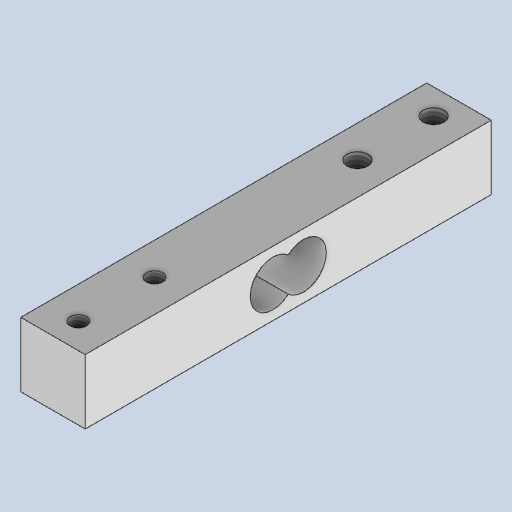
# Autodesk Inventor part: SC133-20kg
Saved by Autodesk Inventor 2022 (Build 260153000, 153)
## iProperties
Part Number: SC133-20kg
Material: 一般
Document SubType Name: Modeling
Designer: Masato Kubotera
Density: 1 g/cm^3
Appearance: 既定
Catalog Web Link: https://akizukidenshi.com/catalog/g/gP-12034/
Description: ReadyMade
Mass: 10.9137 g
Surface Area: 51.8776 cm^2
Volume: 10.9137 cm^3
Author: Masato Kubotera
Autodesk Inventor part; units mm, degrees
ref_plane "YZ Plane" through (0, 0, 0) normal (1, 0, 0) x (0, 1, 0)
ref_plane "XZ Plane" through (0, 0, 0) normal (0, 1, 0) x (-1, 0, 0)
ref_plane "XY Plane" through (0, 0, 0) normal (0, 0, 1) x (1, 0, 0)
sketch "スケッチ1" plane through (0, 0, 0) normal (0, 1, 0) x (-1, 0, 0)
  line L0 (-40, 6.35) -> (40, 6.35)
  line L1 (40, 6.35) -> (40, -6.35)
  line L2 (40, -6.35) -> (-40, -6.35)
  line L3 (-40, -6.35) -> (-40, 6.35)
  line L4 (-40, 6.35) -> (40, -6.35) construction
  line L5 (40, 6.35) -> (-40, -6.35) construction
  arc A0 (0, 3.3541) -> (0, -3.3541) centre (-3, 0) ccw
  line L6 (-40, 0) -> (0, 0) construction
  line L7 (0, 6.35) -> (0, -6.35) construction
  arc A1 (0, -3.3541) -> (0, 3.3541) centre (3, 0) ccw
  point P0 (0, -3.3541)
  dimension "d0" = 80
  dimension "d1" = 12.7
  dimension "d2" = 9
  dimension "d3" = 3
  constraints: 16 end point, 5 midpoint, 4 point on circle, 3 point on line, 3 symmetric about line, 2 centre point, 2 horizontal, 2 parallel, 1 perpendicular, 1 other
  measures "d0" distance of L1.end L2.end
  measures "d1" distance of L0.end L1.end
  measures "d2" diameter of A0
  measures "d3" distance of L6.end A0.centre
extrude "押し出し1" add sketch "スケッチ1" along normal mid plane 12.7
sketch "スケッチ2" plane through (-40, 6.35, 6.35) normal (0, 0, 1) x (1, 0, 0)
  line L0 (80, -12.7) -> (80, 0) projected
  line L1 (80, -6.35) -> (0, -6.35) construction
  line L2 (0, -12.7) -> (0, 0) projected
  line L3 (80, 0) -> (0, 0) projected
  line L4 (40, 0) -> (40, -12.7) construction
  line L5 (80, -12.7) -> (0, -12.7) projected
  point P0 (40, -6.35)
  point P1 (75, -6.35)
  point P2 (60, -6.35)
  point P3 (20, -6.35)
  point P4 (5, -6.35)
  dimension "d6" = 15
  dimension "d7" = 15
  dimension "d8" = 40
  constraints: 4 end point, 4 midpoint, 4 point on line, 1 symmetric about line
  measures "d6" distance of point (60, -6.35) point (75, -6.35)
  measures "d7" distance of point (5, -6.35) point (20, -6.35)
  measures "d8" distance of point (20, -6.35) point (60, -6.35)
hole "穴1" at (35, 0, 6.35) at (20, 0, 6.35) direction (0, 0, -1) diameter 3.242 end through all thread size "M4x0.7" class "6H" standard "ISO Metric profile"
hole "穴2" at (-20, 0, 6.35) at (-35, 0, 6.35) direction (0, 0, -1) diameter 4.134 end through all thread size "M5x0.8" class "6H" standard "ISO Metric profile"
